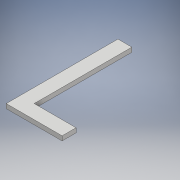
# Autodesk Inventor part: Liu_Inital_L
Saved by Autodesk Inventor 2017 (Build 210142000, 142)
## iProperties
Created: 2016-09-28
Part Number: Liu_Inital_L
Material: Generic
Document SubType Name: Modeling
Designer: jliu
Density: 1 g/cm^3
Appearance: Default
Author: jliu
Autodesk Inventor part; units mm, degrees
ref_plane "YZ Plane" through (0, 0, 0) normal (1, 0, 0) x (0, 1, 0)
ref_plane "XZ Plane" through (0, 0, 0) normal (0, 1, 0) x (-1, 0, 0)
ref_plane "XY Plane" through (0, 0, 0) normal (0, 0, 1) x (1, 0, 0)
sketch "Sketch1" plane through (0, 0, 0) normal (0, 0, 1) x (1, 0, 0)
  line L0 (5, -35) -> (5, 35)
  line L1 (5, 35) -> (-5, 35)
  line L2 (-5, 35) -> (-5, -45)
  line L3 (-5, -45) -> (35, -45)
  line L4 (35, -45) -> (35, -35)
  line L5 (35, -35) -> (5, -35)
  point P0 (0, 0)
  dimension "d0" = 10
  dimension "d1" = 35
  dimension "d2" = 80
  dimension "d3" = 35
  dimension "d4" = 5
  dimension "d5" = 40
  constraints: 12 end point, 5 perpendicular, 1 vertical
  measures "d0" distance of L0.end L1.end
  measures "d1" vertical distance of point (0, 0) L0.end
  measures "d2" distance of L2.end L1.end
  measures "d3" vertical distance of L0.start point (0, 0)
  measures "d4" distance from line of L2 point (0, 0)
  measures "d5" distance of L3.end L2.end
extrude "Extrusion1" add sketch "Sketch1" along normal mid plane 3.175
body "Solid1"
